makerbeam-8cm-handle v3 (Autodesk Fusion 360 design; units mm, degrees)
Autodesk Fusion 360 part; units mm, degrees
box "BoxPrimitive1" add length 60 width 120 height 15 placed x (0, 0, -1) y (-1, 0, 0) z (0, 1, 0) at (120, 0, 0)
fillet "Fillet1" radius 20 1 edges at (0, 7.5, -60)
fillet "Fillet1" radius 20 1 edges at (120, 7.5, -60)
box "BoxPrimitive2" cut length 10.2 width 10.1 height -120 placed x (0, 1, 0) y (0, 0, 1) z (1, 0, 0) at (120, 2.4, -10.1)
box "BoxPrimitive3" cut length 30 width 80 height -60 placed x (0, 0, -1) y (-1, 0, 0) z (0, 1, 0) at (100, 15, -20)
fillet "Fillet2" radius 8 1 edges at (20, 7.5, -50)
fillet "Fillet2" radius 8 1 edges at (100, 7.5, -50)
fillet "Fillet2" radius 8 1 edges at (100, 7.5, -20)
fillet "Fillet2" radius 8 1 edges at (20, 7.5, -20)
cylinder "CylinderPrimitive1" cut diameter 3.1 height -15 placed x (1, 0, 0) y (0, 0, -1) z (0, 1, 0) at (60, 15, -5)
cylinder "CylinderPrimitive2" cut diameter 3.1 height -15 placed x (1, 0, 0) y (0, 0, -1) z (0, 1, 0) at (20, 15, -5)
cylinder "CylinderPrimitive3" cut diameter 3.1 height -15 placed x (1, 0, 0) y (0, 0, -1) z (0, 1, 0) at (100, 15, -5)
fillet "Fillet3" radius 3 8 edges at (60, 15, -50) (22.3431, 15, -47.6569) (20, 15, -35) (22.3431, 15, -22.3431) (60, 15, -20) (97.6569, 15, -22.3431) (100, 15, -35) (97.6569, 15, -47.6569)
fillet "Fillet3" radius 3 8 edges at (97.6569, 0, -47.6569) (60, 0, -50) (22.3431, 0, -47.6569) (20, 0, -35) (22.3431, 0, -22.3431) (60, 0, -20) (97.6569, 0, -22.3431) (100, 0, -35)
fillet "Fillet4" radius 1 1 edges at (120, 13.8, 0)
fillet "Fillet4" radius 1 1 edges at (120, 1.2, 0)
fillet "Fillet4" radius 1 1 edges at (0, 13.8, 0)
fillet "Fillet4" radius 1 1 edges at (0, 1.2, 0)
